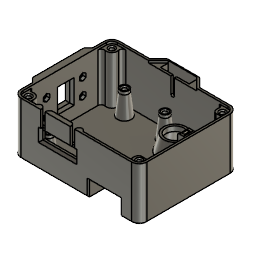
MainCaseBottom (Autodesk Fusion 360 design; units mm, degrees)
Autodesk Fusion 360 part; units mm, degrees
sketch "Skizze1" plane through (0, 0, 0) normal (0, 0, 1) x (1, 0, 0)
  line L0 (50.5, 45) -> (-50.5, 45)
  line L1 (-50.5, -45) -> (50.5, -45)
  line L2 (57.5, -38) -> (57.5, 38)
  line L3 (57.5, 45) -> (-57.5, -45) construction
  line L4 (-57.5, 45) -> (57.5, -45) construction
  line L5 (-61.5, 23.5) -> (-61.5, -23.5)
  line L6 (-61.5, -23.5) -> (-57.5, -27.5)
  line L7 (-61.5, 23.5) -> (-57.5, 27.5)
  line L8 (-61.5, 0) -> (-57.5, 0) construction
  arc A0 (-50.5, 45) -> (-57.5, 38) centre (-50.5, 38) ccw
  arc A1 (-57.5, -38) -> (-50.5, -45) centre (-50.5, -38) ccw
  arc A2 (57.5, 38) -> (50.5, 45) centre (50.5, 38) ccw
  arc A3 (50.5, -45) -> (57.5, -38) centre (50.5, -38) ccw
  line L9 (-55.5, 38) -> (-55.5, -38)
  arc A4 (-55.5, -38) -> (-50.5, -43) centre (-50.5, -38) ccw
  line L10 (-50.5, -43) -> (50.5, -43)
  arc A5 (50.5, -43) -> (55.5, -38) centre (50.5, -38) ccw
  line L11 (55.5, -38) -> (55.5, 38)
  arc A6 (55.5, 38) -> (50.5, 43) centre (50.5, 38) ccw
  line L12 (50.5, 43) -> (-50.5, 43)
  arc A7 (-50.5, 43) -> (-55.5, 38) centre (-50.5, 38) ccw
  line L13 (-57.5, 38) -> (-57.5, 27.5)
  line L14 (-57.5, -27.5) -> (-57.5, -38)
  circle A8 centre (-50.5, 38) radius 2
  circle A9 centre (-50.5, -38) radius 2
  circle A10 centre (50.5, 38) radius 2
  circle A11 centre (50.5, -38) radius 2
  circle A12 centre (15.5, 29.5) radius 8.25
  circle A13 centre (-35.5, -34.5) radius 2
  circle A14 centre (-35.5, 34.5) radius 4
  circle A15 centre (-35.5, 34.5) radius 2
  circle A16 centre (1.5, -34.5) radius 2
  circle A17 centre (1.5, 34.5) radius 4
  circle A18 centre (1.5, 34.5) radius 2
  line L15 (55.5, 0) -> (-55.5, 0) construction
  arc A19 (45.6588, 39.25) -> (51.75, 33.1588) centre (50.5, 38) ccw
  arc A20 (45.6588, 39.25) -> (42.754, 43) centre (42.754, 40) ccw
  arc A21 (55.5, 30.254) -> (51.75, 33.1588) centre (52.5, 30.254) ccw
  arc A22 (-51.75, 33.1588) -> (-45.6588, 39.25) centre (-50.5, 38) ccw
  arc A23 (-45.6588, -39.25) -> (-51.75, -33.1588) centre (-50.5, -38) ccw
  arc A24 (51.75, -33.1588) -> (45.6588, -39.25) centre (50.5, -38) ccw
  arc A25 (42.754, -43) -> (45.6588, -39.25) centre (42.754, -40) ccw
  arc A26 (51.75, -33.1588) -> (55.5, -30.254) centre (52.5, -30.254) ccw
  arc A27 (-45.6588, -39.25) -> (-42.754, -43) centre (-42.754, -40) ccw
  arc A28 (-55.5, -30.254) -> (-51.75, -33.1588) centre (-52.5, -30.254) ccw
  arc A29 (-51.75, 33.1588) -> (-55.5, 30.254) centre (-52.5, 30.254) ccw
  arc A30 (-42.754, 43) -> (-45.6588, 39.25) centre (-42.754, 40) ccw
  circle A31 centre (-35.5, -34.5) radius 4
  circle A32 centre (1.5, -34.5) radius 4
  line L16 (-22.8284, 45) -> (-14.8284, 53)
  line L17 (-14.8284, 53) -> (14.8284, 53)
  line L18 (14.8284, 53) -> (22.8284, 45)
  line L19 (-13, 45) -> (13, 45)
  line L20 (13, 45) -> (13, 52)
  line L21 (13, 52) -> (-13, 52)
  line L22 (-13, 52) -> (-13, 45)
  line L23 (-22, 43) -> (-13, 52)
  line L24 (13, 52) -> (22, 43)
  circle A33 centre (15.5, 29.5) radius 10.25
  dimension "d1" = 90
  dimension "d2" = 115
  dimension "d3" = 4
  dimension "d4" = 135
  dimension "d5" = 135
  dimension "d6" = 47
  dimension "d7" = 0
  dimension "d8" = 7
  dimension "d9" = 7
  dimension "d10" = 7
  dimension "d11" = 7
  dimension "d19" = 5
  dimension "d20" = 4
  dimension "d21" = 3
  dimension "d22" = 3
  dimension "d23" = 4
  dimension "d24" = 8
  dimension "d25" = 37
  dimension "d26" = 34.5
  dimension "d85" = 16.5
  dimension "d120" = 26
  dimension "d121" = 13
  dimension "d122" = 2
  dimension "d123" = 2
  dimension "d125" = 44
  dimension "d126" = 37
  dimension "d129" = 69
  dimension "d130" = 69
  dimension "d133" = 14
  dimension "d136" = 5
  dimension "d137" = 20.5
  dimension "d138" = 20
  dimension "d232" = 10
  constraint horizontal L0
  constraint perpendicular L0 L13
  constraint parallel L0 L1
  constraint parallel L2 L13
  constraint coincident L3 origin
  constraint coincident L4 origin
  constraint vertical L5
  constraint coincident L6.end L13
  constraint coincident L5 L8.start
  constraint coincident L8.end L13
  constraint perpendicular L8 L13
  constraint symmetric L6 L7 L8
  constraint coincident L4.start L13
  constraint coincident L4.start L0
  constraint tangent A0 L13
  constraint tangent L0 A0
  constraint coincident L3.end L13
  constraint coincident L3.end L1
  constraint tangent A1 L13
  constraint tangent L1 A1
  constraint coincident L3.start L0
  constraint coincident L3.start L2
  constraint tangent L0 A2
  constraint tangent L2 A2
  constraint coincident L4.end L1
  constraint coincident L4.end L2
  constraint tangent L1 A3
  constraint tangent L2 A3
  constraint collinear L13 L14
  constraint concentric A1 A4
  constraint concentric A3 A5
  constraint concentric A2 A6
  constraint concentric A0 A7
  constraint tangent L9 A7
  constraint tangent A4 L10
  constraint tangent L9 A4
  constraint tangent L12 A7
  constraint tangent A6 L12
  constraint tangent L10 A5
  constraint tangent A5 L11
  constraint tangent L11 A6
  constraint coincident origin L15
  constraint horizontal L15
  constraint coincident L11 L15.start
  constraint coincident L9 L15.end
  constraint coincident A2.centre A6.centre
  constraint coincident L12 A20.end
  constraint tangent A19 A20
  constraint coincident L11 A21.start
  constraint tangent A19 A21
  constraint tangent A6 A19
  constraint tangent L11 A21
  constraint tangent L12 A20
  constraint equal A8 A10
  constraint equal A8 A9
  constraint equal A9 A11
  constraint coincident A0.centre A7.centre
  constraint coincident A1.centre A4.centre
  constraint coincident A3.centre A5.centre
  constraint coincident L10 A25.start
  constraint tangent A24 A25
  constraint coincident L11 A26.end
  constraint tangent A24 A26
  constraint coincident L10 A27.end
  constraint tangent A23 A27
  constraint coincident L9 A28.start
  constraint tangent A23 A28
  constraint coincident L9 A29.end
  constraint tangent A22 A29
  constraint coincident L12 A30.start
  constraint tangent A22 A30
  constraint equal A19 A22
  constraint equal A22 A23
  constraint equal A23 A24
  constraint tangent L12 A30
  constraint tangent L9 A29
  constraint tangent L9 A28
  constraint tangent L10 A27
  constraint tangent L10 A25
  constraint tangent L11 A26
  constraint equal A20 A30
  constraint equal A29 A30
  constraint equal A28 A29
  constraint equal A27 A28
  constraint equal A25 A27
  constraint equal A25 A26
  constraint tangent A7 A22
  constraint tangent A4 A23
  constraint tangent A5 A24
  constraint equal A14 A31
  constraint equal A14 A17
  constraint equal A31 A32
  constraint equal A13 A15
  constraint equal A15 A18
  constraint equal A16 A18
  constraint horizontal A13.centre A16.centre
  constraint coincident A16.centre A32.centre
  constraint coincident A13.centre A31.centre
  constraint coincident A14.centre A15.centre
  constraint vertical A13.centre A14.centre
  constraint coincident A17.centre A18.centre
  constraint coincident L0 L16.start
  constraint parallel L0 L17
  constraint coincident L0 L18.end
  constraint perpendicular L16 L18
  constraint horizontal L19
  constraint vertical L20
  constraint horizontal L21
  constraint vertical L22
  constraint coincident L0 L19.start
  constraint coincident L12 L23.start
  constraint coincident L12 L24.end
  constraint parallel L18 L24
  constraint concentric A12 A33
  measures "d1" distance of L4.start L3.end
  measures "d2" distance of L3.end L4.end
  measures "d3" distance of L5 L13
  measures "d4" angle of L5 L7
  measures "d5" angle of L5 L6
  measures "d6" distance of L5.start L5.end
  measures "d7" distance of origin L8
  measures "d8" radius of A0
  measures "d9" radius of A1
  measures "d10" radius of A2
  measures "d11" radius of A3
  measures "d19" radius of A19
  measures "d20" diameter of A10
  measures "d21" radius of A21
  measures "d22" radius of A20
  measures "d23" diameter of A13
  measures "d24" diameter of A31
  measures "d25" distance of A13.centre A16.centre
  measures "d26" vertical distance of origin A14.centre
  measures "d85" diameter of A12
  measures "d120" distance of L20 L22
  measures "d121" distance of origin L22
  measures "d122" distance of L16 L23
  measures "d123" distance of L18 L24
  measures "d125" distance of L23.start L24.end
  measures "d126" distance of A14.centre A17.centre
  measures "d129" distance of A16.centre A17.centre
  measures "d130" distance of A13.centre A14.centre
  measures "d133" horizontal distance of A12.centre A17.centre
  measures "d136" vertical distance of A12.centre A17.centre
  measures "d137" diameter of A33
  measures "d138" distance of L9 A14.centre
  measures "d232" distance of L12 L17
extrude "Extrusion1" add sketch "Skizze1" along normal blind 47 contours L0 L1 L2 L5 L6 L7 A0 A1 A2 A3 L9 A4 L10 A5 L11 A6 L12 A7 L13 L14 L23 L24 | L0 L16 L17 L18 L21 L23 L24 makes body 1
extrude "Extrusion2" add sketch "Skizze1" against normal blind 1 separate body contours L0 L1 L2 L5 L6 L7 A0 A1 A2 A3 L9 A4 L10 A5 L11 A6 L12 A7 L13 L14 L23 L24 | L0 L16 L17 L18 L21 L23 L24 | L0 L12 L19 L23 L24 | L0 L20 L24 | L0 L19 L20 L21 L22 | L9 L10 L11 L12 A19 A20 A21 A22 A23 A24 A25 A26 A27 A28 A29 A30 | L0 L22 L23 | L11 A6 L12 A19 A20 A21 | L9 L12 A7 A22 A29 A30 | L10 A5 L11 A24 A25 A26 | L9 A4 L10 A23 A27 A28 | A8 | A9 | A10 | A11 | A13 | A14 | A15 | A16 | A17 | A18 | A31 | A32 | A33 makes body 2
extrude "Extrusion3" add sketch "Skizze1" along normal blind 45 contours L0 L12 L19 L23 L24 | L0 L20 L24 | L0 L22 L23 | L11 A6 L12 A19 A20 A21 | L9 L12 A7 A22 A29 A30 | L10 A5 L11 A24 A25 A26 | L9 A4 L10 A23 A27 A28 bodies 1 2
extrude "Extrusion28" add 1 faces at (-4.3333, 47.3333, 0) along direction (0, 0, 1) blind 10 on bodies 1 bodies 1
extrude "Extrusion4" add sketch "Skizze1" along normal blind 30 contours A8 | A9 | A10 | A11 bodies 1
extrude "Extrusion5" add sketch "Skizze1" along normal blind 1 contours L9 L10 L11 L12 A19 A20 A21 A22 A23 A24 A25 A26 A27 A28 A29 A30 | L11 A6 L12 A19 A20 A21 | L9 L12 A7 A22 A29 A30 | L10 A5 L11 A24 A25 A26 | L9 A4 L10 A23 A27 A28 | A8 | A9 | A10 | A11 | A13 | A14 | A15 | A16 | A17 | A18 | A31 | A32 bodies 1
extrude "Extrusion25" add sketch "Skizze1" along normal blind 15 contours A33 bodies 1
draft "Verjüngung2" angle 16 neutral plane through (0, 0, 15) pull (0, 0, 1) 1 faces at (25.6991, 28.4794, 5.6667) on bodies 1
extrude "Extrusion6" add sketch "Skizze1" against normal blind 20 draft 7 from surface at 20 contours A13 | A14 | A15 | A16 | A17 | A18 | A31 | A32 bodies 1
extrude "Extrusion7" add sketch "Skizze1" along normal blind 2.7 from surface at 20 contours A14 | A17 | A31 | A32 bodies 1
extrude "Extrusion8" cut sketch "Skizze1" against normal blind 9 from surface at 20 contours A13 | A15 | A16 | A18 bodies 1
chamfer "Fase2" distance 1 angle 45 8 edges at (-37.3647, -33.7768, 22.7) (-0.3647, -33.7768, 22.7) (-0.3647, 35.2232, 22.7) (-37.3647, 35.2232, 22.7) (-52.3647, 38.7232, 45) (-52.3647, -37.2768, 45) (48.6353, -37.2768, 45) (48.6353, 38.7232, 45) on bodies 1
sketch "Skizze2" plane through (0, 0, 0) normal (0, 1, 0) x (1, 0, 0)
  line L0 (-32.5, -30) -> (-1.5, -30)
  line L1 (-1.5, -30) -> (-1.5, -22)
  line L2 (-1.5, -22) -> (-32.5, -22)
  line L3 (-32.5, -22) -> (-32.5, -30)
  line L4 (-32.5, -26) -> (-1.5, -26) construction
  line L5 (-20, -30.5) -> (20, -30.5) construction
  line L6 (20, -30.5) -> (20, -15.5) construction
  line L7 (20, -15.5) -> (-20, -15.5) construction
  line L8 (-20, -15.5) -> (-20, -30.5) construction
  line L9 (20, -23) -> (-20, -23) construction
  line L10 (0.5, -47) -> (-34.5, -47)
  line L11 (-34.5, -47) -> (-34.5, -20)
  line L12 (-34.5, -20) -> (0.5, -20)
  line L13 (0.5, -20) -> (0.5, -47)
  line L14 (-1.5, -30) -> (-28.5, -30)
  line L15 (-34.5, -20) -> (0.5, -20)
  line L16 (0.5, -20) -> (0.5, -32)
  line L17 (0.5, -32) -> (-34.5, -32)
  line L18 (-34.5, -32) -> (-34.5, -20)
  line L19 (-36.5, -18) -> (2.5, -18)
  line L20 (2.5, -18) -> (2.5, -47)
  line L21 (2.5, -47) -> (-36.5, -47)
  line L22 (-36.5, -47) -> (-36.5, -18)
  line L23 (-32.5, -32) -> (-28.5, -32)
  line L24 (-28.5, -32) -> (-28.5, -47)
  line L25 (-28.5, -47) -> (-32.5, -47)
  line L26 (-32.5, -47) -> (-32.5, -32)
  line L27 (-1.5, -32) -> (-5.5, -32)
  line L28 (-5.5, -32) -> (-5.5, -47)
  line L29 (-5.5, -47) -> (-1.5, -47)
  line L30 (-1.5, -47) -> (-1.5, -32)
  dimension "d55" = 31
  dimension "d56" = 8
  dimension "d58" = 26
  dimension "d92" = 8
  dimension "d93" = 15
  dimension "d94" = 40
  dimension "d95" = 23
  dimension "d96" = 20
  dimension "d141" = 1.5
  dimension "d239" = 17
  dimension "d240" = 2
  dimension "d241" = 2
  dimension "d242" = 2
  dimension "d248" = 2
  dimension "d249" = 2
  dimension "d250" = 2
  dimension "d251" = 2
  dimension "d252" = 29
  dimension "d253" = 4
  dimension "d254" = 4
  dimension "d255" = 2
  dimension "d256" = 2
  text T0 "GPS" font "Arial Black" height 8 align centre middle in box 40 x 15 at (-20, -30.5) x (1, 0) y (0, 1) spacing 1 kerned
  constraint horizontal L0
  constraint vertical L1
  constraint horizontal L2
  constraint vertical L3
  constraint midpoint L3 L4.start
  constraint midpoint L1 L4.end
  constraint coincident L9.start
  constraint coincident L9.end
  constraint horizontal L9
  constraint horizontal L10
  constraint vertical L11
  constraint horizontal L12
  constraint vertical L13
  constraint horizontal L14
  constraint horizontal L15
  constraint vertical L16
  constraint horizontal L17
  constraint vertical L18
  constraint coincident L13 L16.end
  constraint horizontal L19
  constraint vertical L20
  constraint horizontal L21
  constraint vertical L22
  constraint horizontal L23
  constraint vertical L24
  constraint horizontal L25
  constraint vertical L26
  constraint coincident L10 L24.end
  constraint coincident L17 L23.start
  constraint horizontal L27
  constraint vertical L28
  constraint horizontal L29
  constraint vertical L30
  constraint coincident L10 L28.end
  constraint coincident L17 L27.start
  measures "d55" distance of L0.start L0.end
  measures "d56" distance of L0.start L2.end
  measures "d58" distance of origin L4
  measures "d95" distance of origin L9
  measures "d96" distance of origin L8
  measures "d141" distance of origin L1
  measures "d239" distance of L0 L10
  measures "d240" distance of L1 L13
  measures "d241" distance of L2 L12
  measures "d242" distance of L3 L11
  measures "d248" distance of L0 L17
  measures "d249" distance of L18 L22
  measures "d250" distance of L12 L19
  measures "d251" distance of L16 L20
  measures "d252" distance of L19 L21
  measures "d253" distance of L24 L26
  measures "d254" distance of L28 L30
  measures "d255" distance of L18 L26
  measures "d256" distance of L13 L30
extrude "Extrusion29" add sketch "Skizze2" along normal blind 2 from surface at -43 contours L10 L13 L17 L21 L30 | L11 L12 L13 L15 L16 L18 L19 L20 L21 L22 | L11 L12 L13 L15 L16 L17 L18 L23 L27 | L10 L17 L21 L24 L28 | L10 L11 L17 L21 L26 bodies 1
extrude "Extrusion9" cut sketch "Skizze2" against normal blind 2 from surface at -43 contours L0 L1 L2 L3 L14 | L10 L17 L21 L27 L28 L29 L30 | L11 L12 L13 L15 L16 L17 L18 L23 L27 | L10 L17 L21 L23 L24 L25 L26 bodies 1
chamfer "Fase3" distance 2 angle 45 11 edges at (-32.5, -41, 39.5) (-28.5, -41, 39.5) (-5.5, -41, 39.5) (-1.5, -41, 39.5) (-17, -43, 18) (2.5, -43, 32.5) (-36.5, -43, 32.5) (0.5, -43, 26) (-17, -43, 20) (-34.5, -43, 26) (-17, -43, 32) on bodies 1
sketch "Skizze3" plane through (0, 0, 0) normal (1, 0, 0) x (0, 1, 0)
  circle A0 centre (16.5, 15.5) radius 1.75
  circle A1 centre (16.5, 30.5) radius 1.75
  circle A2 centre (-16.5, 15.5) radius 1.75
  circle A3 centre (-16.5, 30.5) radius 1.75
  line L0 (16.5, 15.5) -> (-16.5, 15.5) construction
  line L1 (-16.5, 15.5) -> (-16.5, 30.5) construction
  line L2 (-16.5, 30.5) -> (16.5, 30.5) construction
  line L3 (16.5, 30.5) -> (16.5, 15.5) construction
  line L4 (0, 15.5) -> (0, 30.5) construction
  line L5 (-19.4, 28.8257) -> (-16.5, 27.1514)
  line L6 (-16.5, 27.1514) -> (-13.6, 28.8257)
  line L7 (-13.6, 28.8257) -> (-13.6, 32.1743)
  line L8 (-13.6, 32.1743) -> (-16.5, 33.8486)
  line L9 (-16.5, 33.8486) -> (-19.4, 32.1743)
  line L10 (-19.4, 32.1743) -> (-19.4, 28.8257)
  line L11 (-13.6, 17.1743) -> (-16.5, 18.8486)
  line L12 (-16.5, 18.8486) -> (-19.4, 17.1743)
  line L13 (-19.4, 17.1743) -> (-19.4, 13.8257)
  line L14 (-19.4, 13.8257) -> (-16.5, 12.1514)
  line L15 (-16.5, 12.1514) -> (-13.6, 13.8257)
  line L16 (-13.6, 13.8257) -> (-13.6, 17.1743)
  line L17 (13.6, 13.8257) -> (16.5, 12.1514)
  line L18 (16.5, 12.1514) -> (19.4, 13.8257)
  line L19 (19.4, 13.8257) -> (19.4, 17.1743)
  line L20 (19.4, 17.1743) -> (16.5, 18.8486)
  line L21 (16.5, 18.8486) -> (13.6, 17.1743)
  line L22 (13.6, 17.1743) -> (13.6, 13.8257)
  line L23 (13.6, 28.8257) -> (16.5, 27.1514)
  line L24 (16.5, 27.1514) -> (19.4, 28.8257)
  line L25 (19.4, 28.8257) -> (19.4, 32.1743)
  line L26 (19.4, 32.1743) -> (16.5, 33.8486)
  line L27 (16.5, 33.8486) -> (13.6, 32.1743)
  line L28 (13.6, 32.1743) -> (13.6, 28.8257)
  line L29 (6.5, 32) -> (-4.5, 32)
  line L30 (-4.5, 32) -> (-4.5, 14)
  line L31 (-4.5, 14) -> (6.5, 14)
  line L32 (6.5, 14) -> (6.5, 32)
  point P0 (-16.5, 30.5)
  point P1 (-16.5, 15.5)
  point P2 (16.5, 15.5)
  point P3 (16.5, 30.5)
  dimension "d65" = 3.5
  dimension "d66" = 33
  dimension "d67" = 15
  dimension "d71" = 15.5
  dimension "d73" = 2.9
  dimension "d74" = 2.9
  dimension "d75" = 2.9
  dimension "d76" = 2.9
  dimension "d106" = 11
  dimension "d107" = 12
  dimension "d108" = 18
  dimension "d109" = 1.5
  dimension "d110" = 1.5
  constraint horizontal L0
  constraint vertical L1
  constraint horizontal L2
  constraint vertical L3
  constraint coincident P0 A3.centre
  constraint coincident P2 A0.centre
  constraint coincident P1 L1
  constraint coincident P3 A1.centre
  constraint equal A0 A2
  constraint equal A1 A3
  constraint equal A0 A1
  constraint coincident P1 A2.centre
  constraint vertical L4
  constraint symmetric L1 L3 L4
  constraint coincident L2 L4.end
  constraint coincident L0 L4.start
  constraint vertical L10
  constraint vertical L28
  constraint vertical L22
  constraint vertical L16
  constraint horizontal L29
  constraint vertical L30
  constraint horizontal L31
  constraint vertical L32
  measures "d65" diameter of A0
  measures "d66" distance of P0 P3
  measures "d67" distance of P1 P0
  measures "d71" distance of L0 origin
  measures "d73" distance of P0 L10
  measures "d74" distance of P1 L16
  measures "d75" distance of P2 L22
  measures "d76" distance of P3 L28
  measures "d106" distance of L30.end L31.end
  measures "d107" horizontal distance of P0 L29.end
  measures "d108" distance of L29.start L31.end
  measures "d109" vertical distance of P0 L29.start
  measures "d110" vertical distance of P1 L31.end
extrude "Extrusion10" cut sketch "Skizze3" along normal up to surface (6 mm away) from surface at -61.5 contours A0 | A1 | A2 | A3 | L29 L30 L31 L32 bodies 1
extrude "Extrusion11" cut sketch "Skizze3" against normal blind 3 from surface at -55.5 contours L5 L6 L7 L8 L9 L10 | L11 L12 L13 L14 L15 L16 | L17 L18 L19 L20 L21 L22 | L23 L24 L25 L26 L27 L28 bodies 1
chamfer "Fase4" distance 2 angle 45 4 edges at (-55.5, 6.5, 23) (-55.5, 1, 32) (-55.5, -4.5, 23) (-55.5, 1, 14) on bodies 1
extrude "Extrusion12" add sketch "Skizze2" along normal blind 0.5 from surface at 53 text T0 bodies 1
sketch "Skizze6" plane through (0, 0, 1) normal (0, 0, 1) x (-1, 0, 0)
  circle A0 centre (-1.5, 34.5) radius 6.3329
  circle A1 centre (35.5, 34.5) radius 6.3329
  circle A2 centre (35.5, -34.5) radius 6.3329
  arc A3 (-55.5, -30.254) -> (-51.75, -33.1588) centre (-52.5, -30.254) ccw
  arc A4 (-45.6588, -39.25) -> (-51.75, -33.1588) centre (-50.5, -38) ccw
  arc A5 (-45.6588, -39.25) -> (-42.754, -43) centre (-42.754, -40) ccw
  line L0 (-10.893, -43) -> (42.754, -43)
  arc A6 (42.754, -43) -> (45.6588, -39.25) centre (42.754, -40) ccw
  arc A7 (51.75, -33.1588) -> (45.6588, -39.25) centre (50.5, -38) ccw
  arc A8 (51.75, -33.1588) -> (55.5, -30.254) centre (52.5, -30.254) ccw
  line L1 (55.5, -30.254) -> (55.5, 30.254)
  arc A9 (55.5, 30.254) -> (51.75, 33.1588) centre (52.5, 30.254) ccw
  arc A10 (45.6588, 39.25) -> (51.75, 33.1588) centre (50.5, 38) ccw
  arc A11 (45.6588, 39.25) -> (42.754, 43) centre (42.754, 40) ccw
  line L2 (42.754, 43) -> (-42.754, 43)
  arc A12 (-42.754, 43) -> (-45.6588, 39.25) centre (-42.754, 40) ccw
  arc A13 (-51.75, 33.1588) -> (-45.6588, 39.25) centre (-50.5, 38) ccw
  arc A14 (-51.75, 33.1588) -> (-55.5, 30.254) centre (-52.5, 30.254) ccw
  line L3 (-55.5, 30.254) -> (-55.5, -30.254)
  line L4 (-55.5, -43) -> (-33.5, -43)
  line L5 (-33.5, -43) -> (-33.5, 43)
  line L6 (-33.5, 43) -> (-55.5, 43)
  line L7 (-55.5, 43) -> (-55.5, -43)
  line L8 (-33.5, -34) -> (-55.5, -34)
  line L9 (-55.5, -34) -> (-55.5, 34)
  line L10 (-55.5, 34) -> (-33.5, 34)
  line L11 (-33.5, 34) -> (-33.5, -34)
  arc A15 (-5.3532, -39.5258) -> (-1.2977, -28.1703) centre (-1.5, -34.5) ccw
  arc A16 (-10.893, -43) -> (-5.3532, -39.5258) centre (-15.5, -29.5) ccw
  line L12 (-42.754, -43) -> (-20.107, -43)
  arc A17 (-1.2977, -28.1703) -> (-20.107, -43) centre (-15.5, -29.5) ccw
  dimension "d142" = 86
  dimension "d143" = 22
  dimension "d144" = 68
  dimension "d145" = 9
  constraint horizontal L4
  constraint vertical L5
  constraint horizontal L6
  constraint vertical L7
  constraint midpoint L3 L7
  constraint horizontal L8
  constraint vertical L9
  constraint horizontal L10
  constraint vertical L11
  constraint coincident L3 L9.end
  constraint coincident L5 L8.start
  measures "d142" distance of L4.end L5.end
  measures "d143" distance of L4.start L4.end
  measures "d144" distance of L8 L10
  measures "d145" distance of L4 L8
extrude "Extrusion13" cut sketch "Skizze6" along normal blind 44 contours A3 A4 L7 L8 L9 | A13 A14 L7 L9 L10 bodies 1
sketch "Skizze7" plane through (0, 0, 0) normal (0, 1, 0) x (1, 0, 0)
  circle A0 centre (40, -29.5) radius 9.5
  circle A1 centre (40, -29.5) radius 11.5
  circle A2 centre (40, -29.5) radius 13.5
  line L0 (55.5, -1) -> (55.5, -45)
  line L1 (55.5, -45) -> (55.5, -47)
  line L2 (55.5, -47) -> (55.5, -45)
  line L3 (55.5, -45) -> (55.5, -1)
  line L4 (5.3532, -1) -> (-4.8329, -1)
  line L5 (7.8329, -1) -> (-4.8329, -1)
  line L6 (-29.1671, -1) -> (-41.8329, -1)
  line L7 (-29.1671, -1) -> (-41.8329, -1)
  line L8 (55.5, -1) -> (47.5, -1)
  line L9 (45.5, -1) -> (47.5, -1)
  line L10 (45.754, -1) -> (42.754, -1)
  line L11 (-42.754, -1) -> (-45.754, -1)
  line L12 (-51.75, -1) -> (-45.5, -1)
  line L13 (-51.75, -1) -> (-55.5, -1)
  line L14 (-51.75, -1) -> (-55.5, -1)
  line L15 (-51.75, -1) -> (-45.5, -1)
  line L16 (-42.754, -1) -> (-45.754, -1)
  line L17 (-42.754, -1) -> (42.754, -1)
  line L18 (45.754, -1) -> (42.754, -1)
  line L19 (45.5, -1) -> (47.5, -1)
  line L20 (47.5, -1) -> (55.5, -1)
  line L21 (55.5, -1) -> (25.5, -1)
  line L22 (25.5, -1) -> (25.5, -43)
  line L23 (25.5, -43) -> (55.5, -43)
  line L24 (55.5, -43) -> (55.5, -1)
  line L25 (55.5, -1) -> (25.5, -1)
  line L26 (25.5, -1) -> (25.5, -24)
  line L27 (25.5, -24) -> (55.5, -24)
  line L28 (55.5, -24) -> (55.5, -1)
  line L29 (55.5, -1) -> (53.5, -1)
  line L30 (53.5, -1) -> (53.5, -43)
  line L31 (53.5, -43) -> (55.5, -43)
  line L32 (55.5, -43) -> (55.5, -1)
  line L33 (40, -29.5) -> (55.5, -29.5)
  line L34 (55.5, -29.5) -> (55.5, -1)
  line L35 (55.5, -1) -> (40, -1)
  line L36 (40, -1) -> (40, -29.5)
  line L37 (42.754, -1) -> (20.107, -1)
  line L38 (29.7644, -1) -> (1.2977, -1)
  line L39 (10.893, -1) -> (5.3532, -1)
  line L40 (10.893, -1) -> (-42.754, -1)
  point P0 (40, -29.5)
  dimension "d148" = 19
  dimension "d149" = 23
  dimension "d150" = 27
  dimension "d151" = 15.5
  dimension "d157" = 2
  dimension "d159" = 30
  dimension "d160" = 42
  dimension "d225" = 13.5
  dimension "d226" = 19
  constraint coincident P0 A0.centre
  constraint concentric A0 A1
  constraint horizontal L21
  constraint vertical L22
  constraint horizontal L23
  constraint vertical L24
  constraint coincident L0.start L3.end
  constraint horizontal L25
  constraint vertical L26
  constraint horizontal L27
  constraint vertical L28
  constraint coincident L22 L26.end
  constraint horizontal L29
  constraint vertical L30
  constraint horizontal L31
  constraint vertical L32
  constraint coincident L23 L30.end
  constraint horizontal L33
  constraint vertical L34
  constraint horizontal L35
  constraint vertical L36
  measures "d148" diameter of A0
  measures "d149" diameter of A1
  measures "d150" diameter of A2
  measures "d151" horizontal distance of P0 L0.end
  measures "d157" distance of L1.end L30
  measures "d159" distance of L22.end L23.end
  measures "d160" distance of L0.start L23.end
  measures "d225" distance of L23 L33
  measures "d226" distance of L23 L27
extrude "Extrusion14" add sketch "Skizze7" along normal blind 9 from surface at 22 contours A0 A1 L27 L33 | A0 A1 L27 L36 | A0 A1 L27 L36 | A1 A2 L27 L33 | A1 A2 L27 L36 | A1 A2 L27 L36 | A2 L27 L30 | L0 L3 L24 L27 L30 L32 L33 L34 | A2 L8 L9 L10 L17 L18 L19 L20 L21 L25 L27 L30 L35 L36 L37 | A2 L17 L21 L22 L25 L26 L27 L36 L37 L38 | L0 L3 L8 L20 L21 L24 L25 L27 L28 L29 L30 L32 L34 L35 picked at (49.723, -24.7648) picked at (52.003, -25.0237) bodies 1
extrude "Extrusion15" cut sketch "Skizze7" along normal blind 5 from surface at 24 contours A1 A2 L27 L33 | A1 A2 L27 L36 | A1 A2 L27 L36 picked at (52.003, -25.0237) bodies 1
extrude "Extrusion16" add sketch "Skizze7" against normal blind 9 from surface at -22 contours A0 A1 L27 L33 | A0 A1 L27 L36 | A0 A1 L27 L36 | A1 A2 L27 L33 | A1 A2 L27 L36 | A1 A2 L27 L36 | A2 L27 L30 | L0 L3 L24 L27 L30 L32 L33 L34 | A2 L8 L9 L10 L17 L18 L19 L20 L21 L25 L27 L30 L35 L36 L37 | A2 L17 L21 L22 L25 L26 L27 L36 L37 L38 | L0 L3 L8 L20 L21 L24 L25 L27 L28 L29 L30 L32 L34 L35 picked at (49.723, -24.7648) picked at (52.003, -25.0237) bodies 1
extrude "Extrusion17" cut sketch "Skizze7" against normal blind 5 from surface at -24 contours A1 A2 L27 L33 | A1 A2 L27 L36 | A1 A2 L27 L36 picked at (52.003, -25.0237) bodies 1
sketch "Skizze8" plane through (0, 43, 0) normal (0, -1, 0) x (1, 0, 0)
  line L0 (20.107, 1) -> (42.754, 1)
  line L1 (42.754, 1) -> (42.754, 45)
  line L2 (42.754, 45) -> (50.5, 45)
  line L3 (50.5, 45) -> (50.5, 47)
  line L4 (50.5, 47) -> (22, 47)
  line L5 (22, 47) -> (22, 45)
  line L6 (22, 45) -> (-22, 45)
  line L7 (-22, 45) -> (-22, 47)
  line L8 (-50.5, 47) -> (-50.5, 45)
  line L9 (-50.5, 45) -> (-42.754, 45)
  line L10 (-42.754, 45) -> (-42.754, 1)
  line L11 (-1.5, 45) -> (1.5, 45)
  line L12 (1.5, 45) -> (1.5, 29)
  line L13 (1.5, 29) -> (-1.5, 29)
  line L14 (-1.5, 29) -> (-1.5, 45)
  spline S0 degree 2 poles (10.893, 1) (15.5, 6.1889) (20.107, 1) knots 0 0 0 1.06454 1.06454 1.06454 weights 1 1.056625 1
  line L15 (-42.754, 1) -> (10.893, 1)
  line L16 (-22, 47) -> (-50.5, 47)
  dimension "d181" = 3
  dimension "d182" = 16
  constraint horizontal L11
  constraint vertical L12
  constraint horizontal L13
  constraint vertical L14
  constraint midpoint L6 L11
  measures "d181" distance of L12.end L13.end
  measures "d182" distance of L11.start L13.end
extrude "Extrusion18" cut sketch "Skizze8" against normal blind 2 contours L6 L11 L12 L13 L14 bodies 1
fillet "Abrundung2" radius 1.5 6 edges at (49.5, 26.5, 29.5) (25.5, 26.5, 24) (49.5, -26.5, 29.5) (25.5, -26.5, 24) (1.5, 44, 29) (-1.5, 44, 29) on bodies 1
fillet "Abrundung2" radius 2.5 4 edges at (47.5, -34, 23) (47.5, 34, 23) (32.254, -26.5, 24) (32.254, 26.5, 24) on bodies 1
fillet "Abrundung2" radius 3 2 edges at (55.5, -34, 23) (55.5, 34, 23) on bodies 1
sketch "Skizze9" plane through (0, 0, 1) normal (0, 0, 1) x (-1, 0, 0)
  circle A0 centre (35.5, -34.5) radius 6.3329
  circle A1 centre (35.5, 34.5) radius 6.3329
  circle A2 centre (-1.5, 34.5) radius 6.3329
  line L0 (-10.893, -43) -> (42.754, -43)
  arc A3 (42.754, -43) -> (45.6588, -39.25) centre (42.754, -40) ccw
  arc A4 (51.75, -33.1588) -> (45.6588, -39.25) centre (50.5, -38) ccw
  arc A5 (51.75, -33.1588) -> (55.5, -30.254) centre (52.5, -30.254) ccw
  line L1 (55.5, -30.254) -> (55.5, 30.254)
  arc A6 (55.5, 30.254) -> (51.75, 33.1588) centre (52.5, 30.254) ccw
  arc A7 (45.6588, 39.25) -> (51.75, 33.1588) centre (50.5, 38) ccw
  arc A8 (45.6588, 39.25) -> (42.754, 43) centre (42.754, 40) ccw
  line L2 (42.754, 43) -> (-42.754, 43)
  arc A9 (-42.754, 43) -> (-45.6588, 39.25) centre (-42.754, 40) ccw
  arc A10 (-46.5, 35) -> (-45.6588, 39.25) centre (-50.5, 38) ccw
  line L3 (-55.5, 31) -> (-25.5, 31)
  line L4 (-25.5, 31) -> (-25.5, 22)
  line L5 (-25.5, 22) -> (-55.5, 22)
  line L6 (-55.5, 22) -> (-55.5, -22)
  line L7 (-55.5, -22) -> (-27.6336, -22)
  line L8 (-9, 43) -> (-42, 43)
  line L9 (-42, 43) -> (-42, 22)
  line L10 (-42, 22) -> (-9, 22)
  line L11 (-9, 22) -> (-9, 43)
  line L12 (-11, 27) -> (-40, 27)
  line L13 (-40, 27) -> (-40, 43)
  line L14 (-40, 43) -> (-11, 43)
  line L15 (-11, 43) -> (-11, 27)
  line L16 (-42, 22) -> (-17, 22)
  arc A11 (-5.3532, -39.5258) -> (-1.2977, -28.1703) centre (-1.5, -34.5) ccw
  arc A12 (-1.2977, -28.1703) -> (-27.6336, -22) centre (-15.5, -29.5) ccw
  line L17 (-17, 22) -> (-34, 22)
  line L18 (-34, 22) -> (-34, 0)
  line L19 (-34, 0) -> (-17, 0)
  line L20 (-17, 0) -> (-17, 22)
  arc A13 (-10.893, -43) -> (-5.3532, -39.5258) centre (-15.5, -29.5) ccw
  arc A14 (-52.5, 34) -> (-55.5, 31) centre (-52.5, 31) ccw
  arc A15 (-48.5, 34) -> (-46.5, 35) centre (-48.5, 36.5) ccw
  line L21 (-48.5, 34) -> (-52.5, 34)
  dimension "d185" = 21
  dimension "d186" = 33
  dimension "d187" = 7.5
  dimension "d188" = 2
  dimension "d189" = 2
  dimension "d190" = 5
  dimension "d216" = 17
  dimension "d217" = 22
  dimension "d218" = 8
  constraint horizontal L8
  constraint vertical L9
  constraint horizontal L10
  constraint vertical L11
  constraint coincident L2 L8.start
  constraint horizontal L12
  constraint vertical L13
  constraint horizontal L14
  constraint vertical L15
  constraint coincident L8 L13.end
  constraint horizontal L16
  constraint horizontal L17
  constraint vertical L18
  constraint horizontal L19
  constraint vertical L20
  measures "d185" distance of L8.end L9.end
  measures "d186" distance of L9.end L10.end
  measures "d187" distance of A2.centre L11
  measures "d188" distance of L9 L13
  measures "d189" distance of L11 L15
  measures "d190" distance of L10 L12
  measures "d216" distance of L18.end L19.end
  measures "d217" distance of L17.end L18.end
  measures "d218" distance of L9 L18
extrude "Extrusion19" cut sketch "Skizze9" against normal blind 2 contours L2 L3 L4 L8 L12 L13 L14 L15 | L3 L4 L12 L13 bodies 1
extrude "Extrusion20" add sketch "Skizze9" along normal blind 12 contours L3 L4 L5 L9 L10 L12 L13 L16 L17 | L2 L3 L8 L9 L13 | L2 L4 L8 L10 L11 L12 L15 L16 L17 bodies 1
sketch "Skizze10" plane through (0, 0, 13) normal (0, 0, 1) x (-1, 0, 0)
  line L0 (-11, 43) -> (-11, 27)
  line L1 (-11, 27) -> (-25.5, 27)
  line L2 (-25.5, 22) -> (-9, 22)
  line L3 (-9, 43) -> (-42, 43)
  line L4 (-42, 43) -> (-42, 22)
  line L5 (-42, 22) -> (-9, 22)
  line L6 (-9, 22) -> (-9, 43)
  line L7 (-9, 43) -> (-11, 43)
  line L8 (-9, 22) -> (-9, 43)
  line L9 (-25.5, 27) -> (-25.5, 22)
  dimension "d229" = 21
  dimension "d231" = 33
  constraint horizontal L3
  constraint horizontal L5
  constraint vertical L6
  constraint coincident L2.end L5.end
  constraint vertical L4
  measures "d229" distance of L3.start L2.end
  measures "d231" distance of L4.end L2.end
extrude "Extrusion21" add sketch "Skizze10" along normal blind 2 bodies 1
extrude "Extrusion22" cut 1 faces at (20.6667, -43, 3.6667) along direction (0, -1, 0) blind 2 on bodies 1 bodies 1
extrude "Extrusion27" cut 1 faces at (35.1667, -28.3333, 1) along direction (0, 0, 1) blind 12 on bodies 1 bodies 1
sketch "Skizze11" plane through (0, -27, 0) normal (0, -1, 0) x (1, 0, 0)
  line L0 (11, 13) -> (11, -1)
  line L1 (11, -1) -> (40, -1)
  line L2 (40, -1) -> (40, 13)
  line L3 (40, 13) -> (11, 13)
  circle A0 centre (25.5, 6) radius 3.5
  dimension "d199" = 14.5
  dimension "d200" = 7
  dimension "d201" = 7
  measures "d199" distance of L0 A0.centre
  measures "d200" distance of L3 A0.centre
  measures "d201" diameter of A0
extrude "Extrusion23" cut sketch "Skizze11" against normal blind 5 contours A0 bodies 1
chamfer "Fase6" distance 1 angle 45 20 edges at (55.4497, -42.9497, -1) (57.5, 0, -1) (55.4497, 42.9497, -1) (36.6642, 45, -1) (45.25, -45, -1) (-57.5, -32.75, -1) (-55.4497, -42.9498, -1) (-19.75, -45, -1) (-36.6642, 45, -1) (-55.4497, 42.9497, -1) (-57.5, 32.75, -1) (-59.5, -25.5, -1) (-59.5, 25.5, -1) (-61.5, 0, -1) (-18.8284, 49, -1) (0, 53, -1) (18.8284, 49, -1) (25.5, -45, 13) (11, -45, 6) (40, -45, 6) on bodies 1
fillet "Abrundung3" radius 2 3 edges at (42, -37, 15) (9, -32.5, 15) (25.5, -26.5, 15) on bodies 1
chamfer "Fase7" distance 4 distance2 11.5 1 edges at (7.8083, 26.5167, -1) measured on face at (-34.7722, 8.2842, -1) on bodies 1
equation "d25 = mount_dx"
equation "d26 = mount_dy / 2"
equation "d72 = d7"
equation "d109 = d110"
equation "d126 = mount_dx"
equation "mount_dx = 37 mm"
equation "mount_dy = 69 mm"
equation "d129 = mount_dy"
equation "d130 = mount_dy"
equation "d133 = ultrasonic_dx"
equation "d136 = ultrasonic_dy"
equation "ultrasonic_dx = 14 mm"
equation "ultrasonic_dy = 5 mm"
equation "d235 = us_cone_diameter"
equation "d236 = us_cone_height"
equation "us_cone_diameter = 4 mm"
equation "us_cone_height = 11.5 mm"
